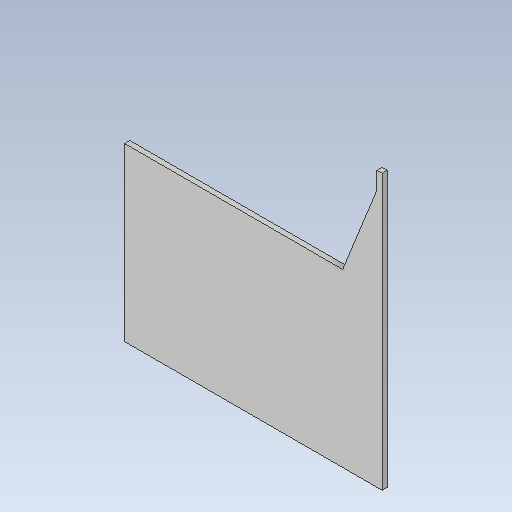
# Autodesk Inventor part: Porton
Saved by Autodesk Inventor 2020 (Build 240168000, 168)
## iProperties
Created: 2020-03-13
Part Number: Porton
Material: Genérico
Document SubType Name: Modeling
Designer: Diego Guillén
Density: 1 g/cm^3
Appearance: Valor por defecto
Author: Diego Guillén
Autodesk Inventor part; units mm, degrees
ref_plane "YZ Plane" through (0, 0, 0) normal (1, 0, 0) x (0, 1, 0)
ref_plane "XZ Plane" through (0, 0, 0) normal (0, 1, 0) x (-1, 0, 0)
ref_plane "XY Plane" through (0, 0, 0) normal (0, 0, 1) x (1, 0, 0)
sketch "Boceto1" plane through (0, 0, 0) normal (0, 0, 1) x (1, 0, 0)
  line L0 (0, 0) -> (150, 0)
  line L1 (150, 0) -> (150, 100)
  line L2 (150, 100) -> (0, 100)
  line L3 (0, 100) -> (0, 0)
  dimension "d0" = 150
  dimension "d1" = 100
  constraints: 8 end point, 2 parallel, 1 horizontal, 1 perpendicular
  measures "d0" distance of L2.end L1.end
  measures "d1" distance of L0.end L1.end
extrude "Extrusión1" add sketch "Boceto1" along normal blind 3
sketch "Boceto2" plane through (0, 100, 0) normal (0, 1, 0) x (1, 0, 0)
  line L0 (150, 0) -> (0, 0) construction
  line L1 (0, 0) -> (0, -3) construction
  line L2 (150, -3) -> (0, -3) construction
  line L3 (150, 0) -> (150, -3) construction
  line L4 (150, 0) -> (147, 0)
  line L5 (147, 0) -> (147, -3)
  line L6 (147, -3) -> (150, -3)
  line L7 (150, -3) -> (150, 0)
  line L8 (150, 0) -> (150, -3) construction
  line L9 (150, -3) -> (0, -3) construction
  point P0 (0, 0)
  dimension "d4" = 3
  dimension "d5" = 3
  constraints: 8 end point, 2 collinear, 2 parallel, 1 horizontal, 1 perpendicular
  measures "d4" distance of L4.end L5.end
  measures "d5" distance of L4.start L4.end
extrude "Extrusión2" add sketch "Boceto2" along normal blind 60
sketch "Boceto3" plane through (0, 0, 3) normal (0, 0, 1) x (1, 0, 0)
  line L0 (0, 0) -> (150, 0) construction
  line L1 (150, 0) -> (150, 160) construction
  line L2 (147, 160) -> (150, 160) construction
  line L3 (147, 100) -> (147, 160) construction
  line L4 (147, 100) -> (0, 100) construction
  line L5 (0, 100) -> (0, 0) construction
  line L6 (147, 100) -> (127, 100)
  line L7 (147, 100) -> (0, 100) construction
  line L8 (127, 100) -> (147, 150)
  line L9 (147, 100) -> (147, 160) construction
  line L10 (147, 150) -> (147, 100)
  dimension "d8" = 20
  dimension "d9" = 10
  constraints: 6 end point, 2 point on line, 1 collinear
  measures "d8" distance of L3.start L6.end
  measures "d9" distance of L2.start L8.end
extrude "Extrusión3" add sketch "Boceto3" against normal blind 3
